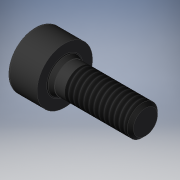
# Autodesk Inventor part: M3x8_p3
Saved by Autodesk Inventor 2019 (Build 230136000, 136)
## iProperties
Created: 2024-03-05
Part Number: M3x8_p3
Material: Generic
Catalog Web Link: www.cadenas.de
Description: MBRDC, MBRDAC_part3-Pulleys for Round Belts - Clemping Type - Trapezoid Groove
Vendor: MISUMI
Document SubType Name: Modeling
Designer: psAdmin
Manufacturer: MISUMI
Mass: 0.116395 g
Surface Area: 1.85217 cm^2
Volume: 0.116395 cm^3
Density: 1 g/cm^3
Appearance: PSOLRGB-175-175-175
Category: PARTsolutions
Company: MISUMI
Title: M3x8
Author: Cadenas PARTsolutions
Comments: Pulleys for Round Belts - Clemping Type - Trapezoid Groove
PSOL_IDENT_0: {$CADENAS_DATA/23d-libs/misumi/metric/52_belts_pulleys/mbrdc/mbrdc_part3.prj},165 {VTYP=3D},{NB=M3x8
PSOL_IDENT_1: _p3},{LINA=M3x8},{NN=MBRDC, MBRDAC_part3},{DATE=06.06.2021 23:11:25},{GEOMDATE=10.06.2016 02:58:32},
PSOL_IDENT_2: {VERSION=},{LINEID=300},{WBVAR=},{WBNUMERIC=}  {NB=M3x8_p3},{LINA=M3x8},{KT=DUMMY},{PN=M3x8},{D=3.00
PSOL_IDENT_3: 0},{D3=2.387},{P=0.500},{L=8.000},{S=2.500},{HM=8.000},{DK=5.500},{DA=3.600},{DS=3.000},{E=2.870},{K=
PSOL_IDENT_4: 3.000},{R=0.100},{T=1.300},{V=0.300},{DW=5.070},{W=1.150},{LF=0.510},{LG=1.500},{FORM=1.000}
NB: M3x8_p3
NN: MBRDC, MBRDAC_part3
NT: Pulleys for Round Belts - Clemping Type - Trapezoid Groove
NBSYN: $PN._p3
LINA: M3x8
CATALOG: Misumi
PN: M3x8
D: 3
D3: 2.387
P: 0.5
L: 8
S: 2.5
HM: 8
DK: 5.5
DA: 3.6
DS: 3
E: 2.87
K: 3
R: 0.1
T: 1.3
V: 0.3
DW: 5.07
W: 1.15
LF: 0.51
LG: 1.5
FORM: 1
SUPPLIER: MISUMI
ARTICLENO: M3x8_p3
BOMINFO: M3x8
CREATOR: CADENAS GmbH
Autodesk Inventor part; units mm, degrees
sketch "Skizze_2" plane through (0, 0, 0) normal (0, 0, 1) x (1, 0, 0)
  line L0 (8, 0) -> (-6, 0)
  line L1 (-0.4283, 0) -> (-1.15, 1.25)
  line L2 (-1.15, 1.25) -> (-2.815, 1.25)
  line L3 (-2.815, 1.25) -> (-3, 1.435)
  line L4 (-3, 1.435) -> (-3, 2.45)
  arc A0 (-2.7, 2.75) -> (-3, 2.45) centre (-2.7, 2.45) ccw
  line L5 (-2.7, 2.75) -> (0, 2.75)
  line L6 (0, 2.75) -> (0, 1.8)
  arc A1 (0, 1.8) -> (0.0562, 1.7101) centre (0.1, 1.8) ccw
  line L7 (0.0562, 1.7101) -> (0.4662, 1.5101)
  arc A2 (0.4662, 1.5101) -> (0.51, 1.5) centre (0.51, 1.6) ccw
  line L8 (0.51, 1.5) -> (7.6935, 1.5)
  line L9 (7.6935, 1.5) -> (8, 1.1935)
  line L10 (8, 1.1935) -> (8, 0)
  line L11 (8, 0) -> (-0.4283, 0)
  constraints: 24 end point, 6 point on circle, 3 centre point
revolve "Revolution1" add sketch "Skizze_2" angle 360 about axis through (8, 0, 0) along (1, 0, 0)
thread "Thread1" size "M3x0.5" class "6g" standard "ISO Metric profile" length 6.1935
sketch "Skizze_1" plane through (-1.15, 0, 0) normal (1, 0, 0) x (0, 0, -1)
  line L0 (-1.25, -0.7217) -> (0, -1.4434)
  line L1 (0, -1.4434) -> (1.25, -0.7217)
  line L2 (1.25, -0.7217) -> (1.25, 0.7217)
  line L3 (1.25, 0.7217) -> (0, 1.4434)
  line L4 (0, 1.4434) -> (-1.25, 0.7217)
  line L5 (-1.25, 0.7217) -> (-1.25, -0.7217)
  constraints: 12 end point
extrude "Extrusion1" cut sketch "Skizze_1" against normal blind 2.6
ref_plane "IP1_XY" through (0, 0, 0) normal (1, 0, 0) x (0, 0, -1)
ref_plane "IP1_YZ" through (0, 0, 0) normal (0, 0, -1) x (0, 1, 0)
ref_plane "IP1_ZX" through (0, 0, 0) normal (0, 1, 0) x (1, 0, 0)
ref_plane "IP2_XY" through (-3, 0, 0) normal (1, 0, 0) x (0, 0, -1)
ref_plane "IP2_YZ" through (-3, 0, 0) normal (0, 0, -1) x (0, 1, 0)
ref_plane "IP2_ZX" through (-3, 0, 0) normal (0, 1, 0) x (1, 0, 0)
ref_plane "IP3_XY" through (8, 0, 0) normal (1, 0, 0) x (0, 0, -1)
ref_plane "IP3_YZ" through (8, 0, 0) normal (0, 0, -1) x (0, 1, 0)
ref_plane "IP3_ZX" through (8, 0, 0) normal (0, 1, 0) x (1, 0, 0)
body "Solid1"
